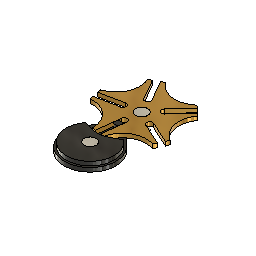
Geneva Wheel Mechanism v1 (Autodesk Fusion 360 design; units mm, degrees)
Autodesk Fusion 360 part; units mm, degrees
note: some values were not read from the file. Set by a fixed rule: which sketch regions a step uses.
sketch "Sketch1" plane through (0, 0, 0) normal (0, 0, 1) x (1, 0, 0) in component "Follower"
  line L0 (0, 0) -> (29.3893, -40.4508) construction
  line L1 (0, 0) -> (50, 0) construction
  line L2 (0, 0) -> (-9.5515, -13.1465) construction
  line L3 (0, 0) -> (50, 0) construction
  line L4 (8.7219, -18.3845) -> (26.3554, -42.655)
  line L5 (32.4231, -38.2467) -> (14.7895, -13.9761)
  arc A0 (14.7895, -13.9761) -> (8.7219, -18.3845) centre (11.7557, -16.1803) ccw
  line L6 (20.1799, 2.6139) -> (48.5777, 11.8409)
  arc A1 (17.8623, 9.7468) -> (20.1799, 2.6139) centre (19.0211, 6.1803) ccw
  line L7 (46.394, 19.0173) -> (17.8623, 9.7468)
  line L8 (3.75, 20) -> (3.75, 50)
  arc A2 (-3.75, 20) -> (3.75, 20) centre (0, 20) ccw
  line L9 (-3.75, 50) -> (-3.75, 20)
  line L10 (-17.8623, 9.7468) -> (-46.394, 19.0173)
  arc A3 (-20.1799, 2.6139) -> (-17.8623, 9.7468) centre (-19.0211, 6.1803) ccw
  line L11 (-48.7116, 11.8844) -> (-20.1799, 2.6139)
  line L12 (-14.7895, -13.9761) -> (-32.4231, -38.2467)
  arc A4 (-8.7219, -18.3845) -> (-14.7895, -13.9761) centre (-11.7557, -16.1803) ccw
  line L13 (-26.3554, -42.655) -> (-8.7219, -18.3845)
  circle A5 centre (0, 0) radius 7.5
  arc A6 (22.1872, -44.8077) -> (-22.1872, -44.8077) centre (0, -65) ccw
  arc A7 (-29.3183, -40.5023) -> (-18.1729, -31.3928) centre (0, -65) ccw construction
  arc A8 (-29.3893, -40.4508) -> (-29.3183, -40.5023) centre (0, 0) ccw
  arc A9 (-26.2727, -42.5411) -> (-22.1872, -44.8077) centre (0, 0) ccw
  arc A10 (22.1872, -44.8077) -> (26.2727, -42.5411) centre (0, 0) ccw
  arc A11 (29.3183, -40.5023) -> (29.3893, -40.4508) centre (0, 0) ccw
  arc A12 (49.4709, 7.2549) -> (35.7584, -34.9476) centre (61.8187, -20.0861) ccw
  arc A13 (8.3875, 49.2915) -> (44.2871, 23.2089) centre (38.206, 52.5861) ccw
  arc A14 (-44.2871, 23.2089) -> (-8.3875, 49.2915) centre (-38.206, 52.5861) ccw
  arc A15 (-35.7584, -34.9476) -> (-49.4709, 7.2549) centre (-61.8187, -20.0861) ccw
  arc A16 (-48.5777, 11.8409) -> (-49.4709, 7.2549) centre (0, 0) ccw
  arc A17 (-35.7584, -34.9476) -> (-32.3403, -38.1327) centre (0, 0) ccw
  arc A18 (-3.75, 49.8592) -> (-8.3875, 49.2915) centre (0, 0) ccw
  arc A19 (-44.2871, 23.2089) -> (-46.2601, 18.9738) centre (0, 0) ccw
  arc A20 (46.2601, 18.9738) -> (44.2871, 23.2089) centre (0, 0) ccw
  arc A21 (8.3875, 49.2915) -> (3.75, 49.8592) centre (0, 0) ccw
  arc A22 (32.3403, -38.1327) -> (35.7584, -34.9476) centre (0, 0) ccw
  arc A23 (50, 0) -> (48.5777, 11.8409) centre (0, 0) ccw
  dimension "d1" = 100
  dimension "d2" = 54
  dimension "d3" = 50
  dimension "d4" = 126
  dimension "d5" = 65
  dimension "d6" = 60
  dimension "d8" = 20
  dimension "d11" = 15
  dimension "d13" = 360
  constraint coincident L0.start L1.start
  constraint horizontal L1
  constraint horizontal L3
  constraint tangent L0 A7
  constraint tangent L2 A7
  constraint concentric A6 A7
  constraint parallel L4 L5
  constraint tangent L5 A0
  constraint tangent L4 A0
  constraint coincident L0 A0.centre
  constraint concentric A5 A10
  constraint coincident L12 A17.end
  constraint concentric A8 A10
  constraint coincident A4 L2.end
  constraint coincident L13 A7.end
  constraint coincident L13 A9.start
  constraint concentric A8 A9
  constraint coincident L10 A19.end
  constraint coincident L11 A16.start
  constraint concentric A10 A16
  constraint coincident L8 A21.end
  constraint coincident L9 A18.start
  constraint concentric A10 A18
  constraint coincident L7 A20.start
  constraint concentric A10 A20
  constraint coincident L5 A22.start
  constraint concentric A10 A22
  constraint coincident L4 A10.end
  constraint coincident A7 A11.start
  constraint concentric A10 A11
  constraint concentric A16 A17
  constraint concentric A18 A19
  constraint concentric A20 A21
  constraint concentric A22 A23
  measures "d1" diameter of A10
  measures "d2" angle of L0 L1
  measures "d3" distance of L0.start L0.end
  measures "d4" angle of L2 L3
  measures "d5" distance of L0.start A6.centre
  measures "d6" diameter of A6
  measures "d8" distance of L0.start A0.centre
  measures "d11" diameter of A5
extrude "Extrude1" add sketch "Sketch1" along normal blind 5 makes body 1 in component "Follower"
sketch "Sketch1 (2)" plane through (0, 0, 0) normal (0, 0, 1) x (1, 0, 0) in component "Cam"
  arc A0 (-29.3183, -40.5023) -> (-18.1729, -31.3928) centre (0, -65) ccw
  circle A1 centre (0, -65) radius 30
  circle A2 centre (0, -65) radius 32.5
  circle A3 centre (0, -65) radius 7.5
  circle A4 centre (0, -26.794) radius 3.75
  line L0 (-24.6979, -43.875) -> (-3.7997, -19.4423)
  line L1 (3.7997, -19.4423) -> (24.6979, -43.875)
  arc A5 (3.7997, -19.4423) -> (-3.7997, -19.4423) centre (0, -22.6923) ccw
  spline S0 degree 2 poles (-22.3607, -45) (0, -53.1337) (20.6252, -43.2146) knots 0 0 0 4.511642 4.511642 4.511642 weights 1 3 1
  point P0 (0, -15)
  dimension "d16" = 60
  dimension "d17" = 65
  dimension "d18" = 15
  dimension "d19" = 7.5
  dimension "d20" = 15
  dimension "d21" = 5
  dimension "d23" = 20
  constraint concentric A0 A1
  constraint concentric A1 A2
  constraint concentric A0 A3
  constraint coincident A0 A4.centre
  constraint coincident A2 L0.start
  constraint coincident A2 L1.end
  constraint tangent A2 L0
  constraint tangent A2 L1
  constraint vertical origin P0
  constraint coincident P0 L0
  constraint coincident P0 L1
  constraint tangent L0 A5
  constraint tangent L1 A5
  constraint coincident A1 S0.end
  constraint coincident A1 S0.start
  measures "d16" diameter of A1
  measures "d17" diameter of A2
  measures "d18" diameter of A3
  measures "d19" diameter of A4
  measures "d20" distance of origin P0
  measures "d21" radius of A5
  measures "d23" distance of A0.centre S0.start
extrude "Extrude1'" add sketch "Sketch1 (2)" against normal blind 5 separate body contours A0 A2 A4 L0 L1 | A0 A4 L0 L1 A5 | A0 A4 | A0 A4 | A2 | A1 S0 | A1 S0 makes body 2 in component "Cam"
extrude "Extrude2" add sketch "Sketch1 (2)" along normal blind 5 contours A0 A4 | A0 A4 | A1 S0 picked at (14.8588, -54.2841) bodies 2 in component "Cam"
cylinder "CylinderPrimitive1" add diameter 15 height -20 placed x (1, 0, 0) y (0, 1, 0) z (0, 0, 1) at (0, 0, 5) separate body makes body 3 in component "Component"
component "Follower" placed x (0.869606, 0.493747, 0) y (-0.493747, 0.869606, 0) z (0, 0, 1) at (0, 0, 0)
component "Cam" placed x (0.996861, 0.079176, 0) y (-0.079176, 0.996861, 0) z (0, 0, 1) at (-5.1464, -0.2041, 0)
component "Component" placed x (1, 0, 0) y (0, 1, 0) z (0, 0, 1) at (0, 0, 0)
component "Component" placed x (1, 0, 0) y (0, 1, 0) z (0, 0, 1) at (0, -65, 0)
